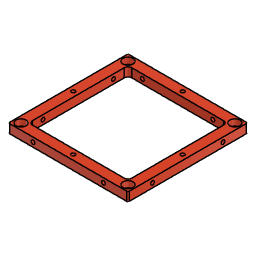
base-holder (Autodesk Fusion 360 design; units mm, degrees)
Autodesk Fusion 360 part; units mm, degrees
sketch "Sketch1" plane through (0, 0, 0) normal (0, 0, 1) x (1, 0, 0)
  line L0 (19, -25) -> (-74, -25)
  line L1 (-75, -24) -> (-75, 69)
  line L2 (-74, 70) -> (19, 70)
  line L3 (20, 69) -> (20, -24)
  arc A0 (-74, 70) -> (-75, 69) centre (-74, 69) ccw
  arc A1 (20, 69) -> (19, 70) centre (19, 69) ccw
  arc A2 (-75, -24) -> (-74, -25) centre (-74, -24) ccw
  arc A3 (19, -25) -> (20, -24) centre (19, -24) ccw
  point P0 (20, -25)
  point P1 (-75, -25)
  point P2 (20, 70)
  dimension "d1" = 95
  dimension "d2" = 95
  dimension "d3" = 1
  constraint horizontal L0
  constraint vertical L1
  constraint horizontal L2
  constraint vertical L3
  constraint tangent L1 A0
  constraint tangent L2 A0
  constraint coincident P2 L2
  constraint coincident P2 L3
  constraint tangent L2 A1
  constraint tangent L3 A1
  constraint equal A0 A1
  constraint coincident P1 L0
  constraint coincident P1 L1
  constraint tangent L0 A2
  constraint tangent L1 A2
  constraint equal A0 A2
  constraint coincident P0 L0
  constraint coincident P0 L3
  constraint tangent L0 A3
  constraint tangent L3 A3
  constraint equal A0 A3
  measures "d1" distance of P0 P1
  measures "d2" distance of P0 P2
  measures "d3" radius of A0
extrude "Extrude1" add sketch "Sketch1" along normal blind 7
sketch "Sketch2" plane through (0, 0, 7) normal (0, 0, 1) x (-1, 0, 0)
  arc A0 (75, 24) -> (74, 25) centre (74, 24) ccw
  line L0 (74, 25) -> (-19, 25)
  arc A1 (-19, 25) -> (-20, 24) centre (-19, 24) ccw
  line L1 (-20, 24) -> (-20, -69)
  arc A2 (-20, -69) -> (-19, -70) centre (-19, -69) ccw
  line L2 (-19, -70) -> (74, -70)
  arc A3 (74, -70) -> (75, -69) centre (74, -69) ccw
  line L3 (75, -69) -> (75, 24)
  line L4 (64, -62) -> (-9, -62)
  line L5 (-12, -59) -> (-12, 14)
  line L6 (-9, 17) -> (64, 17)
  line L7 (67, 14) -> (67, -59)
  arc A4 (64, -62) -> (67, -59) centre (64, -59) ccw
  arc A5 (-12, -59) -> (-9, -62) centre (-9, -59) ccw
  arc A6 (-9, 17) -> (-12, 14) centre (-9, 14) ccw
  arc A7 (67, 14) -> (64, 17) centre (64, 14) ccw
  point P0 (67, -62)
  point P1 (-12, -62)
  point P2 (67, 17)
  dimension "d6" = 79
  dimension "d7" = 79
  dimension "d8" = 3
  dimension "d9" = 8
  dimension "d10" = 8
  constraint horizontal L4
  constraint vertical L5
  constraint horizontal L6
  constraint vertical L7
  constraint coincident P0 L4
  constraint coincident P0 L7
  constraint tangent L4 A4
  constraint tangent L7 A4
  constraint coincident P1 L4
  constraint coincident P1 L5
  constraint tangent L4 A5
  constraint tangent L5 A5
  constraint equal A4 A5
  constraint tangent L5 A6
  constraint tangent L6 A6
  constraint equal A4 A6
  constraint coincident P2 L6
  constraint coincident P2 L7
  constraint tangent L6 A7
  constraint tangent L7 A7
  constraint equal A4 A7
  measures "d6" distance of P0 P1
  measures "d7" distance of P0 P2
  measures "d8" radius of A4
  measures "d9" distance of L2 L4
  measures "d10" distance of L1 L5
extrude "Extrude2" cut sketch "Sketch2" against normal blind 19 contours L4 L5 L6 L7 A4 A5 A6 A7
sketch "Sketch3" plane through (0, 0, 7) normal (0, 0, 1) x (-1, 0, 0)
  line L0 (67, 14) -> (67, -59)
  arc A0 (64, -62) -> (67, -59) centre (64, -59) ccw
  line L1 (64, -62) -> (-9, -62)
  arc A1 (-12, -59) -> (-9, -62) centre (-9, -59) ccw
  line L2 (-12, -59) -> (-12, 14)
  arc A2 (-9, 17) -> (-12, 14) centre (-9, 14) ccw
  line L3 (-9, 17) -> (64, 17)
  arc A3 (67, 14) -> (64, 17) centre (64, 14) ccw
  arc A4 (75, 24) -> (74, 25) centre (74, 24) ccw
  line L4 (74, 25) -> (-19, 25)
  arc A5 (-19, 25) -> (-20, 24) centre (-19, 24) ccw
  line L5 (-20, 24) -> (-20, -69)
  arc A6 (-20, -69) -> (-19, -70) centre (-19, -69) ccw
  line L6 (-19, -70) -> (74, -70)
  arc A7 (74, -70) -> (75, -69) centre (74, -69) ccw
  line L7 (75, -69) -> (75, 24)
  point P0 (27.5, 21)
  point P1 (71, -22.5)
  point P2 (-16, -22.5)
  point P3 (27.5, -66)
  dimension "d13" = 4
  dimension "d14" = 47.5
  dimension "d15" = 4
  dimension "d16" = 47.5
  dimension "d17" = 4
  dimension "d18" = 47.5
  dimension "d19" = 4
  dimension "d20" = 47.5
  measures "d13" distance of L4 P0
  measures "d14" distance of L7 P0
  measures "d15" distance of L7 P1
  measures "d16" distance of L6 P1
  measures "d17" distance of L6 P3
  measures "d18" distance of L7 P3
  measures "d19" distance of L5 P2
  measures "d20" distance of L4 P2
hole "Hole1" at (-27.5, 66, 7) at (16, 22.5, 7) at (-27.5, -21, 7) at (-71, 22.5, 7) direction (0, 0, -1) diameter 3 depth 25 tip angle 118
sketch "Sketch4" plane through (0, -25, 0) normal (0, -1, 0) x (1, 0, 0)
  line L0 (-74, 0) -> (19, 0)
  line L1 (19, 0) -> (19, 7)
  line L2 (19, 7) -> (-74, 7)
  line L3 (-74, 7) -> (-74, 0)
  line L4 (-75, 0) -> (-75, 7)
  point P0 (-27.5, 3.5)
  point P1 (-55.5, 3.5)
  point P2 (0.5, 3.5)
  dimension "d24" = 3.5
  dimension "d25" = 3.5
  dimension "d26" = 3.5
  dimension "d27" = 47.5
  dimension "d28" = 28
  dimension "d29" = 28
  measures "d24" distance of L2 P0
  measures "d25" distance of L2 P1
  measures "d26" distance of L2 P2
  measures "d27" distance of P0 L4
  measures "d28" distance of P0 P1
  measures "d29" distance of P0 P2
hole "Hole2" at (-55.5, -25, 3.5) at (0.5, -25, 3.5) direction (0, 1, 0) diameter 3 depth 124 tip angle 118
sketch "Sketch5" plane through (20, 0, 0) normal (1, 0, 0) x (0, 1, 0)
  line L0 (-24, 0) -> (69, 0)
  line L1 (69, 0) -> (69, 7)
  line L2 (69, 7) -> (-24, 7)
  line L3 (-24, 7) -> (-24, 0)
  line L4 (-25, 0) -> (-25, 7)
  point P0 (-5.5, 3.5)
  point P1 (22.5, 3.5)
  point P2 (50.5, 3.5)
  dimension "d33" = 3.5
  dimension "d34" = 3.5
  dimension "d35" = 3.5
  dimension "d36" = 47.5
  dimension "d37" = 28
  dimension "d38" = 28
  measures "d33" distance of L2 P1
  measures "d34" distance of L2 P0
  measures "d35" distance of L2 P2
  measures "d36" distance of P1 L4
  measures "d37" distance of P0 P1
  measures "d38" distance of P1 P2
hole "Hole3" at (20, -5.5, 3.5) at (20, 50.5, 3.5) direction (-1, 0, 0) diameter 3 depth 124 tip angle 118
sketch "Sketch6" plane through (0, 0, 7) normal (0, 0, 1) x (-1, 0, 0)
  circle A0 centre (27.5, 21) radius 1.5
  circle A1 centre (27.5, -66) radius 1.5
  circle A2 centre (-16, -22.5) radius 1.5
  circle A3 centre (71, -22.5) radius 1.5
  line L0 (67, 14) -> (67, -59)
  arc A4 (64, -62) -> (67, -59) centre (64, -59) ccw
  line L1 (64, -62) -> (-9, -62)
  arc A5 (-12, -59) -> (-9, -62) centre (-9, -59) ccw
  line L2 (-12, -59) -> (-12, 14)
  arc A6 (-9, 17) -> (-12, 14) centre (-9, 14) ccw
  line L3 (-9, 17) -> (64, 17)
  arc A7 (67, 14) -> (64, 17) centre (64, 14) ccw
  arc A8 (75, 24) -> (74, 25) centre (74, 24) ccw
  line L4 (74, 25) -> (-19, 25)
  arc A9 (-19, 25) -> (-20, 24) centre (-19, 24) ccw
  line L5 (-20, 24) -> (-20, -69)
  arc A10 (-20, -69) -> (-19, -70) centre (-19, -69) ccw
  line L6 (-19, -70) -> (74, -70)
  arc A11 (74, -70) -> (75, -69) centre (74, -69) ccw
  line L7 (75, -69) -> (75, 24)
  point P0 (70, 20)
  point P1 (-15, 20)
  point P2 (70, -65)
  point P3 (-15, -65)
  dimension "d42" = 5
  dimension "d43" = 5
  dimension "d44" = 5
  dimension "d45" = 5
  dimension "d46" = 5
  dimension "d47" = 5
  dimension "d48" = 5
  dimension "d49" = 5
  measures "d42" distance of L7 P0
  measures "d43" distance of L4 P0
  measures "d44" distance of L4 P1
  measures "d45" distance of L5 P1
  measures "d46" distance of L7 P2
  measures "d47" distance of L6 P2
  measures "d48" distance of L6 P3
  measures "d49" distance of L5 P3
hole "Hole4" at (15, 65, 7) at (-70, 65, 7) at (-70, -20, 7) at (15, -20, 7) direction (0, 0, -1) diameter 3 depth 10 tip angle 118
sketch "Sketch7" plane through (0, 0, 7) normal (0, 0, 1) x (-1, 0, 0)
  circle A0 centre (70, 20) radius 1.5
  circle A1 centre (-15, -65) radius 1.5
  circle A2 centre (70, -65) radius 1.5
  circle A3 centre (-15, 20) radius 1.5
  circle A4 centre (27.5, 21) radius 1.5
  circle A5 centre (27.5, -66) radius 1.5
  circle A6 centre (-16, -22.5) radius 1.5
  circle A7 centre (71, -22.5) radius 1.5
  line L0 (67, 14) -> (67, -59)
  arc A8 (64, -62) -> (67, -59) centre (64, -59) ccw
  line L1 (64, -62) -> (-9, -62)
  arc A9 (-12, -59) -> (-9, -62) centre (-9, -59) ccw
  line L2 (-12, -59) -> (-12, 14)
  arc A10 (-9, 17) -> (-12, 14) centre (-9, 14) ccw
  line L3 (-9, 17) -> (64, 17)
  arc A11 (67, 14) -> (64, 17) centre (64, 14) ccw
  arc A12 (75, 24) -> (74, 25) centre (74, 24) ccw
  line L4 (74, 25) -> (-19, 25)
  arc A13 (-19, 25) -> (-20, 24) centre (-19, 24) ccw
  line L5 (-20, 24) -> (-20, -69)
  arc A14 (-20, -69) -> (-19, -70) centre (-19, -69) ccw
  line L6 (-19, -70) -> (74, -70)
  arc A15 (74, -70) -> (75, -69) centre (74, -69) ccw
  line L7 (75, -69) -> (75, 24)
  circle A16 centre (70, -65) radius 4
  circle A17 centre (-15, -65) radius 4
  circle A18 centre (70, 20) radius 4
  circle A19 centre (-15, 20) radius 4
  dimension "d53" = 8
  dimension "d54" = 8
  dimension "d55" = 8
  dimension "d56" = 8
  constraint concentric A2 A16
  constraint concentric A1 A17
  constraint concentric A0 A18
  constraint concentric A3 A19
  measures "d53" diameter of A16
  measures "d54" diameter of A17
  measures "d55" diameter of A18
  measures "d56" diameter of A19
extrude "Extrude3" cut sketch "Sketch7" against normal blind 5 contours A16 | A17 | A18 | A19
